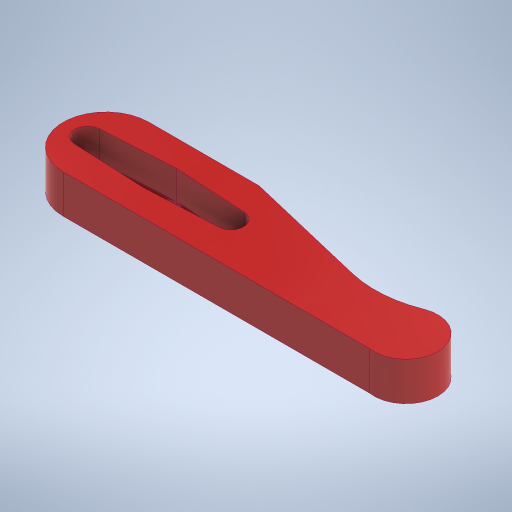
# Autodesk Inventor part: patanueva
Saved by Autodesk Inventor 2024.3 (Build 283343000, 343)
## iProperties
Created: 2025-08-09
Part Number: patanueva
Material: Generic
Document SubType Name: Modeling
Designer: jscme
Density: 1 g/cm^3
Appearance: Pink
Author: jscme
Autodesk Inventor part; units mm, degrees
ref_plane "YZ Plane" through (0, 0, 0) normal (1, 0, 0) x (0, 1, 0)
ref_plane "XZ Plane" through (0, 0, 0) normal (0, 1, 0) x (-1, 0, 0)
ref_plane "XY Plane" through (0, 0, 0) normal (0, 0, 1) x (1, 0, 0)
sketch "Sketch1" plane through (0, 0, 0) normal (0, 1, 0) x (-1, 0, 0)
  line L0 (-3.0181, -8.89) -> (-25.8781, -8.89)
  line L1 (-3.0181, 8.89) -> (-27.578, 8.89)
  line L2 (-25.8781, -8.89) -> (-51.2781, -2.8161)
  line L3 (-27.578, 8.89) -> (-53.0779, 8.89)
  arc A0 (-51.2781, -2.8161) -> (-65.0775, -3.8214) centre (-56.5948, -25.0493) ccw
  line L4 (-53.0779, 8.89) -> (-66.5181, 8.89)
  arc A1 (-66.5181, 8.89) -> (-65.0775, -3.8214) centre (-67.5384, 2.337) ccw
  arc A2 (-3.0181, -8.89) -> (-3.0181, 8.89) centre (-3.0181, 0) ccw
  point P0 (0, 0)
  point P1 (-74.1281, 1.5902)
  point P2 (5.8719, 0)
  dimension "d31" = 80
  dimension "d32" = 8.89
  dimension "d33" = 6.6319
  dimension "d35" = 25.4
  dimension "d36" = 63.5
  dimension "d37" = 22.86
  dimension "d38" = 22.86
  constraints: 10 end point, 8 point on circle, 4 horizontal, 4 tangent, 3 centre point, 1 horizontal alignment
  measures "d31" horizontal distance of point (-74.128, 1.59) point (5.872, 0)
  measures "d32" radius of A2
  measures "d33" radius of A1
  measures "d35" horizontal distance of L0.end L2.end
  measures "d36" distance of L4.end L1.start
  measures "d37" distance of L0.start L0.end
  measures "d38" radius of A0
extrude "Extrusion1" add sketch "Sketch1" along normal blind 8
sketch "Sketch3" plane through (0, 8, 0) normal (0, 1, 0) x (1, 0, 0)
  circle A0 centre (14.1281, 0) radius 3.429
  arc A1 (3.0181, 8.89) -> (3.0181, -8.89) centre (3.0181, 0) ccw projected
  line L0 (14.1281, 3.429) -> (-0.8719, 2.5603)
  line L1 (14.1281, -3.429) -> (-0.8805, -2.725)
  arc A2 (-0.8719, 2.5603) -> (-0.8805, -2.725) centre (-0.7188, -0.0826) ccw
  line L2 (14.1281, 5.8203) -> (14.1281, -4.2261)
  line L3 (14.1281, 3.429) -> (29.1281, 2.5603)
  line L4 (14.1281, -3.429) -> (29.1368, -2.725)
  arc A3 (29.1368, -2.725) -> (29.1281, 2.5603) centre (28.9751, -0.0826) ccw
  circle A4 centre (7.6311, -0.0783) radius 0.75
  circle A5 centre (3.6311, -0.0783) radius 0.75
  circle A6 centre (-0.3689, -0.0783) radius 0.75
  circle A7 centre (20.6252, -0.0783) radius 0.75
  circle A8 centre (24.6252, -0.0783) radius 0.75
  circle A9 centre (28.6252, -0.0783) radius 0.75
  point P0 (-5.8719, 0)
  point P1 (-5.8719, 0)
  point P2 (14.1281, 0.7971)
  point P3 (25.2381, 0)
  point P4 (14.4491, -3.4139)
  point P5 (14.524, 3.4061)
  point P6 (13.7323, 3.4061)
  point P7 (13.8072, -3.4139)
  point P8 (1.1225, -0.0783)
  point P9 (-3.3661, -0.0783)
  dimension "d40" = 20
  dimension "d41" = 15
  dimension "d42" = 15.0086
  dimension "d43" = 6
  dimension "d56" = 6.858
  dimension "d57" = 6
  dimension "d58" = 1.5
  dimension "d59" = 1.5
  dimension "d60" = 1.5
  dimension "d61" = 4
  dimension "d62" = 4
  dimension "d64" = 2.9972
  constraints: 10 end point, 9 centre point, 9 point on circle, 8 symmetric about line, 5 horizontal alignment, 3 vertical alignment, 1 equal length, 1 midpoint, 1 tangent, 1 vertical, 4 other
  measures "d40" distance of point (-5.872, 0) A0.centre
  measures "d41" horizontal distance of L0.start L0.end
  measures "d42" horizontal distance of L1.start L1.end
  measures "d43" angle of L1 L0
  measures "d56" diameter of A0
  measures "d57" angle of L4 L3
  measures "d58" diameter of A6
  measures "d59" diameter of A5
  measures "d60" diameter of A4
  measures "d61" distance of A6.centre A5.centre
  measures "d62" distance of A5.centre A4.centre
  measures "d64" distance of point (-3.366, -0.078) A6.centre
extrude "Extrusion2" cut sketch "Sketch3" against normal through all contours L2 L3 A0 | A0 L0 L2
extrude "Extrusion3" cut sketch "Sketch3" against normal blind 6 contours L1 A2 L0 A0 | A0 L3 A3 L4 | A4 | A5 | A6 | A7 | A8 | A9
sketch "Sketch5" plane through (0, 8, 0) normal (0, 1, 0) x (1, 0, 0)
  circle A0 centre (7.6311, -0.0783) radius 0.75
  circle A1 centre (3.6311, -0.0783) radius 0.75
  circle A2 centre (-0.3689, -0.0783) radius 0.75
  arc A3 (-0.8719, 2.5603) -> (-0.8805, -2.725) centre (-0.7188, -0.0826) ccw projected
  line L0 (14.1281, 12.8466) -> (14.1281, -5.9886)
  circle A4 centre (20.6252, -0.0783) radius 0.75
  circle A5 centre (24.6252, -0.0783) radius 0.75
  circle A6 centre (28.6252, -0.0783) radius 0.75
  point P0 (0, 0)
  point P1 (5.5545, -1.8442)
  point P2 (1.8249, -1.9269)
  point P3 (3.6589, -0.0783)
  point P4 (-3.3661, -0.0783)
  point P5 (-3.3661, -0.0783)
  point P6 (14.1281, 3.429)
  point P7 (14.1281, 3.429)
  dimension "d65" = 1.5
  dimension "d66" = 1.5
  dimension "d67" = 1.5
  dimension "d68" = 4
  dimension "d69" = 4
  dimension "d70" = 2.9972
  constraints: 6 centre point, 4 horizontal alignment, 3 symmetric about line, 2 end point, 2 point on circle, 1 coincident, 1 midpoint, 1 vertical, 3 other
  measures "d65" diameter of A2
  measures "d66" diameter of A1
  measures "d67" diameter of A0
  measures "d68" distance of A2.centre A1.centre
  measures "d69" distance of A1.centre A0.centre
  measures "d70" distance of point (-3.366, -0.078) A2.centre
extrude "Extrusion5" cut sketch "Sketch5" against normal blind 25.4
body "Solid1"
